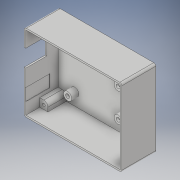
# Autodesk Inventor part: case_bottom
Saved by Autodesk Inventor 2019 (Build 230136000, 136)
## iProperties
Created: 2019-03-24
Part Number: case_bottom
Material: Generic
Document SubType Name: Modeling
Designer: janza
Density: 1 g/cm^3
Appearance: Default
Author: janza
## iProperties of the stored document case_bottom_3DPrint.ipt
Created: 2019-03-26
Part Number: case_bottom_3DPrint
Material: Generic
Document SubType Name: Modeling
Designer: janza
Density: 1 g/cm^3
Appearance: Default
Author: janza
Autodesk Inventor part; units mm, degrees
ref_plane "YZ Plane" through (0, 0, 0) normal (1, 0, 0) x (0, 1, 0)
ref_plane "XZ Plane" through (0, 0, 0) normal (0, 1, 0) x (-1, 0, 0)
ref_plane "XY Plane" through (0, 0, 0) normal (0, 0, 1) x (1, 0, 0)
sketch "Zakladna" plane through (0, 0, 0) normal (0, 0, 1) x (1, 0, 0)
  line L0 (0, 0) -> (92, 0)
  line L1 (92, 0) -> (92, 72)
  line L2 (92, 72) -> (0, 72)
  line L3 (0, 72) -> (0, 0)
  dimension "d0" = 92
  dimension "d1" = 72
  constraints: 8 end point, 2 parallel, 1 horizontal, 1 perpendicular
  measures "d0" distance of L2.end L1.end
  measures "d1" distance of L1.end L0.end
extrude "Extrusion1" add sketch "Zakladna" along normal blind 1.2 and the other way blind 0.4
sketch "Uchyt_arduino" plane through (0, 0, 1.2) normal (0, 0, 1) x (1, 0, 0)
  circle A0 centre (16.2, 12) radius 4
  circle A1 centre (17.2, 60) radius 4
  circle A2 centre (65.5, 44.75) radius 4
  circle A3 centre (65.5, 16.75) radius 4
  circle A4 centre (16.2, 12) radius 4
  circle A5 centre (65.5, 44.75) radius 4
  circle A6 centre (65.5, 16.75) radius 4
  line L0 (0, 72) -> (0, 0) projected
  dimension "d31" = 8
  dimension "d33" = 8
  dimension "d35" = 8
  dimension "d37" = 8
  dimension "d39" = 8
  dimension "d41" = 8
  dimension "d163" = 17.2
  constraints: 7 centre point
  measures "d31" diameter of A0
  measures "d33" diameter of A2
  measures "d35" diameter of A3
  measures "d37" diameter of A4
  measures "d39" diameter of A5
  measures "d41" diameter of A6
  measures "d163" distance from line of L0 A1.centre
sketch "Spojeni_srouby" plane through (0, 0, 1.2) normal (0, 0, 1) x (1, 0, 0)
  line L0 (8, 4) -> (8, 0)
  arc A0 (8, 4) -> (4, 8) centre (4, 4) ccw
  line L1 (4, 8) -> (0, 8)
  line L2 (0, 72) -> (0, 0)
  line L3 (0, 8) -> (0, 0)
  line L4 (0, 0) -> (8, 0)
  line L5 (0, 0) -> (92, 0)
  line L6 (92, 0) -> (92, 36)
  line L7 (92, 0) -> (92, 72)
  line L8 (8, 68) -> (8, 72)
  arc A1 (4, 64) -> (8, 68) centre (4, 68) ccw
  line L9 (4, 64) -> (0, 64)
  line L10 (0, 0) -> (0, 72)
  line L11 (0, 64) -> (0, 72)
  line L12 (0, 72) -> (8, 72)
  line L13 (0, 72) -> (92, 72)
  line L14 (84, 4) -> (84, 0)
  arc A2 (88, 8) -> (84, 4) centre (88, 4) ccw
  line L15 (88, 8) -> (92, 8)
  line L16 (92, 72) -> (92, 0)
  line L17 (92, 8) -> (92, 0)
  line L18 (92, 0) -> (84, 0)
  line L19 (92, 0) -> (0, 0)
  line L20 (84, 68) -> (84, 72)
  arc A3 (84, 68) -> (88, 64) centre (88, 68) ccw
  line L21 (88, 64) -> (92, 64)
  line L22 (92, 0) -> (92, 72)
  line L23 (92, 64) -> (92, 72)
  line L24 (92, 72) -> (84, 72)
  line L25 (92, 72) -> (0, 72)
  constraints: 52 end point, 8 point on circle, 4 centre point, 1 midpoint, 1 perpendicular, 1 vertical
extrude "Extrusion2" add sketch "Uchyt_arduino" along normal blind 7
extrude "Extrusion5" add sketch "Spojeni_srouby" along normal blind 18 contours L0 L4 L2 L1 A0 | L14 A2 L15 L6 L5 | L2 L12 L8 A1 L9 | L21 A3 L20 L13 L7
sketch "diry_srouby" plane through (0, 0, 19.2) normal (0, 0, 1) x (1, 0, 0)
  arc A0 (8, 4) -> (4, 8) centre (4, 4) ccw projected
  arc A1 (88, 8) -> (84, 4) centre (88, 4) ccw projected
  arc A2 (84, 68) -> (88, 64) centre (88, 68) ccw projected
  arc A3 (4, 64) -> (8, 68) centre (4, 68) ccw projected
  point P0 (0, 0)
  constraints: 4 coincident
hole "Hole6" at (4, 4, 19.2) at (88, 4, 19.2) at (88, 68, 19.2) at (4, 68, 19.2) direction (0, 0, -1) diameter 2.8 end through all
sketch "steny" plane through (0, 0, 1.2) normal (0, 0, 1) x (1, 0, 0)
  line L0 (0, 72) -> (0, 56.55)
  line L1 (0, 56.55) -> (-1.6, 56.55)
  line L2 (-1.6, 56.55) -> (-1.6, 72)
  line L3 (-1.6, 72) -> (-1.6, 73.6)
  line L4 (-1.6, 73.6) -> (92, 73.6)
  line L5 (92, 73.6) -> (93.6, 73.6)
  line L6 (93.6, 73.6) -> (93.6, 0)
  line L7 (93.6, 0) -> (93.6, -1.6)
  line L8 (93.6, -1.6) -> (0, -1.6)
  line L9 (0, -1.6) -> (-1.6, -1.6)
  line L10 (-1.6, -1.6) -> (-1.6, 39.75)
  line L11 (-1.6, 39.75) -> (0, 39.75)
  line L12 (0, 0) -> (0, 72) projected
  line L13 (0, 39.75) -> (0, 0)
  line L14 (0, 0) -> (92, 0)
  line L15 (8, 0) -> (84, 0) projected
  line L16 (92, 0) -> (0, 0) projected
  line L17 (92, 0) -> (0, 0)
  line L18 (92, 72) -> (92, 0) projected
  line L19 (0, 0) -> (92, 0)
  line L20 (92, 0) -> (92, 72)
  line L21 (0, 72) -> (92, 72) projected
  line L22 (92, 72) -> (0, 72)
  dimension "d133" = 15.45
  dimension "d134" = 1.6
  dimension "d135" = 1.6
  dimension "d136" = 1.6
  dimension "d137" = 1.6
  dimension "d138" = 1.6
  dimension "d139" = 16.8
  constraints: 36 end point, 7 point on line, 6 perpendicular, 5 collinear, 1 horizontal, 1 vertical
  measures "d133" distance of L0.start L0.end
  measures "d134" distance of L0.end L1.end
  measures "d135" distance of L2.end L3.end
  measures "d136" distance of L4.end L5.end
  measures "d137" distance of L6.end L7.end
  measures "d138" distance of L8.end L9.end
  measures "d139" distance from line of L10.end L1
extrude "Extrusion6" add sketch "steny" along normal blind 31.5 and the other way blind 1.6 contours L0 L1 L2 L3 L4 L5 L6 L7 L8 L9 L10 L11 L12 L14 L18 L21
sketch "stena_RJ45" plane through (0, 0, 1.2) normal (0, 0, 1) x (1, 0, 0)
  line L0 (-1.6, 56.55) -> (0, 56.55) projected
  line L1 (0, 39.75) -> (-1.6, 39.75) projected
  line L2 (-1.6, 39.75) -> (0, 39.75)
  line L3 (0, 56.55) -> (0, 39.75) projected
  line L4 (0, 56.55) -> (0, 39.75)
  line L5 (0, 56.55) -> (-1.6, 56.55)
  line L6 (-1.6, 56.55) -> (-1.6, 39.75)
  line L7 (0, 39.75) -> (-1.6, 39.75)
  point P0 (0, 0)
  constraints: 10 end point, 2 horizontal, 2 perpendicular, 1 collinear
extrude "Extrusion7" add sketch "stena_RJ45" along normal blind 10.9 and the other way blind 1.6
sketch "arduino_uchyt_zavitovaVlozka" plane through (17.2, 60, 8.2) normal (0, 0, 1) x (1, 0, 0)
  circle A0 centre (-1, -48) radius 4 projected
  circle A1 centre (48.3, -43.25) radius 4 projected
  circle A2 centre (48.3, -15.25) radius 4 projected
  circle A3 centre (0, 0) radius 4 projected
  point P0 (-17.2, -60)
  constraints: 4 coincident
hole "Hole7" at (16.2, 12, 8.2) at (65.5, 16.75, 8.2) at (65.5, 44.75, 8.2) at (17.2, 60, 8.2) direction (0, 0, -1) diameter 3.5 depth 7 countersink diameter 3.85 countersink angle 10
sketch "napajeni_znacka1" plane through (-1.6, -1.6, -0.4) normal (-1, 0, 0) x (0, 0, 1)
  circle A0 centre (20.1, 31.85) radius 0.4
  line L0 (12.5, 41.35) -> (33.1, 41.35) projected
  line L1 (0, 0) -> (0, 75.2) projected
  point P0 (0.4, 1.6)
  dimension "d155" = 0.8
  dimension "d156" = 9.5
  dimension "d157" = 20.1
  constraints: 1 centre point
  measures "d155" diameter of A0
  measures "d156" distance from line of L0 A0.centre
  measures "d157" distance from line of L1 A0.centre
ref_plane "napajeni_znacka2_rovina" through (-1.1, -1.6, -0.4) normal (-1, 0, 0) x (0, 0, 1)
sketch "napajeni_znacka2" plane through (-1.1, -1.6, -0.4) normal (-1, 0, 0) x (0, 0, 1)
  point P0 (0.4, 1.6)
  point P1 (20.1, 31.85)
  point P2 (20.1, 31.85)
  constraints: 1 coincident
loft "Loft4" cut profiles "napajeni_znacka1" section 2 point at (-1.1, 30.25, 19.7)
sketch "vyrez_nepouzity_jack" plane through (0, 8, 1.2) normal (1, 0, 0) x (0, 0, -1)
  line L0 (-8, 15.35) -> (-33, 15.35)
  line L1 (-33, 15.35) -> (-33, 3.35)
  line L2 (-33, 3.35) -> (-8, 3.35)
  line L3 (-8, 3.35) -> (-8, 15.35)
  line L4 (-10.9, 31.75) -> (-31.5, 31.75) projected
  line L5 (0, 56) -> (0, 0) projected
  point P0 (1.2, -8)
  dimension "d164" = 25
  dimension "d165" = 12
  dimension "d166" = 16.4
  dimension "d167" = 8
  constraints: 8 end point, 2 parallel, 1 horizontal, 1 perpendicular
  measures "d164" distance of L2.end L1.end
  measures "d165" distance of L1.end L0.end
  measures "d166" distance between parallel lines of L0 L4
  measures "d167" distance between parallel lines of L5 L3
extrude "Extrusion8" cut sketch "vyrez_nepouzity_jack" against normal blind 0.5
fillet "Fillet1" radius 2 4 edges at (-1.6, -1.6, 16.15) (93.6, -1.6, 16.15) (93.6, 73.6, 16.15) (-1.6, 73.6, 16.15)
body "Solid1"
